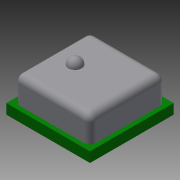
# Autodesk Inventor part: FMA-Sensor-Body
Saved by Autodesk Inventor 2015 (Build 190159000, 159)
## iProperties
Created: 2021-12-01
Part Number: FMA-Sensor-Body
Material: 常规
Document SubType Name: Modeling
Designer: ros
Density: 1 g/cm^3
Appearance: 默认
Author: ros
Autodesk Inventor part; units mm, degrees
ref_plane "YZ Plane" through (0, 0, 0) normal (1, 0, 0) x (0, 1, 0)
ref_plane "XZ Plane" through (0, 0, 0) normal (0, 1, 0) x (-1, 0, 0)
ref_plane "XY Plane" through (0, 0, 0) normal (0, 0, 1) x (1, 0, 0)
sketch "草图1" plane through (0, 0, 0) normal (0, 0, 1) x (1, 0, 0)
  line L0 (-2.5, 2.5) -> (2.5, 2.5)
  line L1 (2.5, 2.5) -> (2.5, -2.5)
  line L2 (2.5, -2.5) -> (-2.5, -2.5)
  line L3 (-2.5, -2.5) -> (-2.5, 2.5)
  point P0 (0, 0)
  point P1 (0, 2.5)
  point P2 (-2.5, 0)
  dimension "d0" = 5
  dimension "d1" = 5
  constraints: 8 end point, 2 midpoint, 2 parallel, 1 horizontal, 1 horizontal alignment, 1 perpendicular, 1 vertical alignment
  measures "d0" distance of L0.start L0.end
  measures "d1" distance of L0.end L1.end
extrude "拉伸1" add sketch "草图1" along normal blind 0.6
sketch "草图2" plane through (0, 0, 0.6) normal (0, 0, 1) x (1, 0, 0)
  line L0 (-2.25, 2.25) -> (2.25, 2.25)
  line L1 (2.25, 2.25) -> (2.25, -2.25)
  line L2 (2.25, -2.25) -> (-2.25, -2.25)
  line L3 (-2.25, -2.25) -> (-2.25, 2.25)
  point P0 (0, 0)
  point P1 (-2.25, 0)
  point P2 (0, 2.25)
  dimension "d4" = 4.5
  dimension "d5" = 4.5
  constraints: 8 end point, 2 midpoint, 2 parallel, 1 horizontal, 1 horizontal alignment, 1 perpendicular, 1 vertical alignment
  measures "d4" distance of L0.start L0.end
  measures "d5" distance of L0.end L1.end
extrude "拉伸2" add sketch "草图2" along normal blind 1.55
sketch "草图3" plane through (0, 0, 2.15) normal (0, 0, 1) x (1, 0, 0)
  line L0 (2.25, 2.25) -> (-2.25, 2.25) projected
  line L1 (-2.25, 2.25) -> (-2.25, -2.25) projected
  line L2 (-2.25, -2.25) -> (2.25, -2.25) projected
  line L3 (2.25, -2.25) -> (2.25, 2.25) projected
  line L4 (2.25, 2.25) -> (2.25, -2.25) projected
  line L5 (2.25, -2.25) -> (-2.25, -2.25) projected
  line L6 (-2.25, -2.25) -> (-2.25, 2.25) projected
  line L7 (-2.25, 2.25) -> (2.25, 2.25) projected
  line L8 (2.5, 2.5) -> (-2.5, 2.5) projected
  line L9 (-2.5, 2.5) -> (-2.5, -2.5) projected
  line L10 (-2.5, -2.5) -> (2.5, -2.5) projected
  line L11 (2.5, -2.5) -> (2.5, 2.5) projected
  arc A0 (-0.49, 0) -> (-1.29, 0) centre (-0.89, 0) ccw
  line L12 (-1.29, 0) -> (-0.49, 0)
  point P0 (0, 0)
  point P1 (-2.25, 0)
  point P2 (-2.5, 0)
  dimension "d8" = 1.61
  dimension "d10" = 0.4
  constraints: 4 horizontal alignment, 2 end point, 2 midpoint, 2 point on circle, 1 centre point, 1 coincident, 1 horizontal
  measures "d8" distance from line of point (-0.89, 0) L9
  measures "d10" radius of A0
revolve "旋转1" add sketch "草图3" angle 360 about axis through (-1.29, 0, 2.15) along (1, 0, 0) contours L12 A0
fillet "圆角1" radius 0.35 4 edges at (-2.25, -2.25, 1.375) (2.25, -2.25, 1.375) (2.25, 2.25, 1.375) (-2.25, 2.25, 1.375)
fillet "圆角2" radius 0.4 8 edges at (-2.1475, 2.1475, 2.15) (-2.25, 0, 2.15) (-2.1475, -2.1475, 2.15) (0, -2.25, 2.15) (2.1475, -2.1475, 2.15) (2.25, 0, 2.15) (2.1475, 2.1475, 2.15) (0, 2.25, 2.15)
equation "\"d1\" = d0"
equation "\"d5\" = d4"
